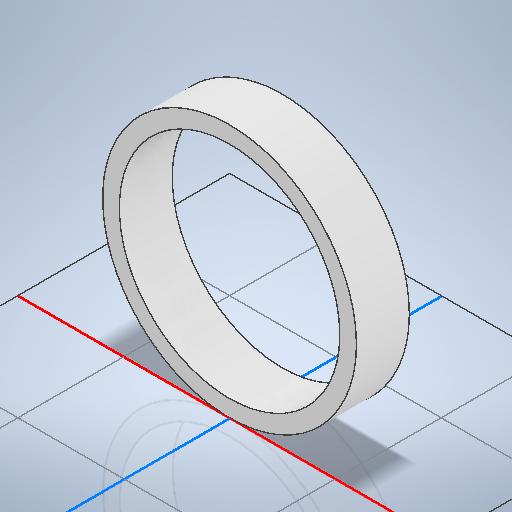
# Autodesk Inventor part: Stretched 2.000 30A .500
Saved by Autodesk Inventor 2026 (Build 300175000, 175)
## iProperties
Created: 2025-04-06
Part Number: Stretched 2.000 30A .500
Material: Rubber, Silicone
Document SubType Name: Modeling
Designer: avere
Density: 1.25 g/cm^3
Appearance: Rubber - Black
Author: avere
Autodesk Inventor part; units mm, degrees
ref_plane "YZ Plane" through (0, 0, 0) normal (1, 0, 0) x (0, 1, 0)
ref_plane "XZ Plane" through (0, 0, 0) normal (0, 1, 0) x (-1, 0, 0)
ref_plane "XY Plane" through (0, 0, 0) normal (0, 0, 1) x (1, 0, 0)
sketch "Sketch1" plane through (0, 0, 0) normal (0, 0, 1) x (1, 0, 0)
  circle A0 centre (0, 0) radius 26.4583
  circle A1 centre (0, 0) radius 30.4583
  dimension "d0" = 4
  constraints: 2 centre point, 2 coincident
  measures "d0" radial gap between concentric circles of A0 A1
extrude "Extrusion1" add sketch "Sketch1" against normal blind 12.7
body "Solid1"
